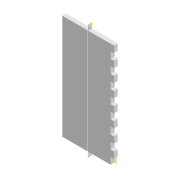
# Autodesk Inventor part: 00_Baseplate_Simmo_side2
Saved by Autodesk Inventor 2022 (Build 260153000, 153)
## iProperties
Created: 2022-05-05
Part Number: 00_Baseplate_Simmo_side2
Material: Generisch
Document SubType Name: Modeling
Designer: diederichbenedict
Density: 1 g/cm^3
Appearance: Vorgabe
Author: diederichbenedict
Autodesk Inventor part; units mm, degrees
ref_plane "YZ Plane" through (0, 0, 0) normal (1, 0, 0) x (0, 1, 0)
ref_plane "XZ Plane" through (0, 0, 0) normal (0, 1, 0) x (-1, 0, 0)
ref_plane "XY Plane" through (0, 0, 0) normal (0, 0, 1) x (1, 0, 0)
ref_plane "Arbeitsebene1" through (0, 0, 0) normal (0, 0, 1) x (1, 0, 0)
sketch "Skizze1" plane through (0, 0, 0) normal (0, 0, 1) x (1, 0, 0)
  circle A0 centre (33, 5) radius 2.95 construction
  line L0 (0, 0) -> (68, 0) construction
  line L1 (68, 0) -> (68, 10) construction
  line L2 (0, 10) -> (68, 10) construction
  line L3 (0, 0) -> (0, 10) construction
  line L4 (68, 10) -> (68, 20) construction
  line L5 (73, 20) -> (73, 10) construction
  line L6 (68, 0) -> (73, 0) construction
  line L7 (73, 10) -> (73, 0) construction
  line L8 (68, 160) -> (73, 160) construction
  line L9 (73, 160) -> (73, 150) construction
  line L10 (-6, 140.2) -> (-6, 149.8) construction
  line L11 (73, 0) -> (-6, 0)
  line L12 (-6, 0) -> (-6, 160)
  line L13 (-6, 160) -> (73, 160)
  line L14 (73, 160) -> (73, 0)
  constraints: 8 end point, 2 parallel, 1 horizontal, 1 perpendicular
extrude "Extrusion1" add sketch "Skizze1" along normal blind 6
sketch "Skizze2" plane through (0, 0, 6) normal (0, 0, -1) x (1, 0, 0)
  line L0 (73, 0) -> (73, -160) projected
  line L1 (68, -10.2) -> (73, -10.2)
  line L2 (73, -10.2) -> (73, 0)
  line L3 (73, 0) -> (68, 0)
  line L4 (68, 0) -> (68, -10.2)
  line L5 (73, -10) -> (68, -10) projected
  line L6 (-6, 0) -> (73, 0) projected
  point P0 (0, 0)
  point P1 (73, 10)
  point P2 (68, 0)
  dimension "d6" = 0.2
  dimension "d7" = 0
  constraints: 8 end point, 2 parallel, 1 horizontal, 1 perpendicular, 1 point on line
  measures "d6" distance between parallel lines of L5 L1
  measures "d7" distance between parallel lines of L6 L3
extrude "Extrusion2" cut sketch "Skizze2" along normal through all
pattern_linear "Rechteckige Anordnung1" count 8 spacing 20 along (0, 1, 0) of "Extrusion2"
ref_plane "Arbeitsebene2" through (33.5, 0, 0) normal (-1, 0, 0) x (0, 0, 1)
